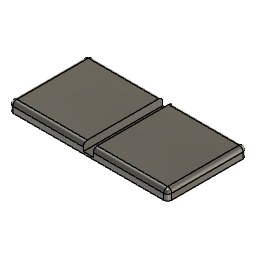
holderbracket v2 (Autodesk Fusion 360 design; units mm, degrees)
Autodesk Fusion 360 part; units mm, degrees
sketch "Sketch1" plane through (0, 0, 0) normal (0, 1, 0) x (1, 0, 0)
  line L0 (-22.5578, -5) -> (57.4422, -5)
  line L1 (57.4422, -5) -> (57.4422, 0)
  line L2 (57.4422, 0) -> (-22.5578, 0)
  line L3 (-22.5578, 0) -> (-22.5578, -5)
  line L4 (14.9422, -5) -> (19.9422, -5)
  line L5 (19.9422, -5) -> (19.9422, -1)
  line L6 (19.9422, -1) -> (14.9422, -1)
  line L7 (14.9422, -1) -> (14.9422, -5)
  dimension "d1" = 5
  dimension "d2" = 80
  dimension "d3" = 5
  dimension "d4" = 4
  dimension "d5" = 37.5
  constraint horizontal L0
  constraint vertical L1
  constraint horizontal L2
  constraint vertical L3
  constraint horizontal L4
  constraint vertical L5
  constraint horizontal L6
  constraint vertical L7
  constraint coincident L0 L4.start
  measures "d1" distance of L0.start L2.end
  measures "d2" distance of L1.end L2.end
  measures "d3" distance of L5.end L6.end
  measures "d4" distance of L4.end L5.end
  measures "d5" distance of L0.start L4.start
extrude "Extrude1" add sketch "Sketch1" along normal blind 40 contours L0 L1 L2 L3 L5 L6 L7
fillet "Fillet1" radius 2 1 edges at (57.4422, 20, 5)
fillet "Fillet2" radius 2 1 edges at (-22.5578, 20, 5)
fillet "Fillet3" radius 2 3 edges at (-22.5578, 0, 1.5) (-21.972, 0, 4.4142) (-2.8078, 0, 5)
fillet "Fillet4" radius 2 3 edges at (37.6922, 0, 5) (56.8564, 0, 4.4142) (57.4422, 0, 1.5)
fillet "Fillet5" radius 2 3 edges at (37.6922, 40, 5) (56.8564, 40, 4.4142) (57.4422, 40, 1.5)
fillet "Fillet6" radius 2 3 edges at (-22.5578, 40, 1.5) (-21.972, 40, 4.4142) (-2.8078, 40, 5)
